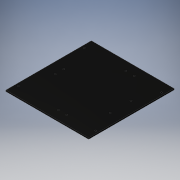
# Autodesk Inventor part: BottomPlate
Saved by Autodesk Inventor 2016 (Build 200138000, 138)
## iProperties
Created: 2015-08-28
Part Number: BottomPlate
Material: Generic
Document SubType Name: Modeling
Designer: lachesis
Density: 1 g/cm^3
Appearance: Glossy - Black
Author: lachesis
Autodesk Inventor part; units mm, degrees
ref_plane "YZ Plane" through (0, 0, 0) normal (1, 0, 0) x (0, 1, 0)
ref_plane "XZ Plane" through (0, 0, 0) normal (0, 1, 0) x (-1, 0, 0)
ref_plane "XY Plane" through (0, 0, 0) normal (0, 0, 1) x (1, 0, 0)
sketch "Block1" plane through (0, 0, 0) normal (0, 0, 1) x (1, 0, 0)
  circle A0 centre (244.9891, 313.0766) radius 1.651
  circle A1 centre (305.4278, 286.7035) radius 1.651
  circle A2 centre (242.5353, 295.4667) radius 1.651
  circle A3 centre (307.8815, 304.3134) radius 1.651
  circle A4 centre (325.7478, 277.8135) radius 1.651
  circle A5 centre (227.9578, 277.8135) radius 1.651
  circle A6 centre (194.5568, 203.1375) radius 1.651
  circle A7 centre (325.7478, 166.5615) radius 1.651
  circle A8 centre (227.9578, 166.5615) radius 1.651
  circle A9 centre (247.0078, 166.5615) radius 1.651
  circle A10 centre (344.7978, 166.5615) radius 1.651
  circle A11 centre (194.5568, 241.2375) radius 1.651
  circle A12 centre (247.0078, 277.8135) radius 1.651
  circle A13 centre (344.7978, 277.8135) radius 1.651
  circle A14 centre (181.8568, 156.6555) radius 1.905
  circle A15 centre (181.8568, 312.8401) radius 1.905
  circle A16 centre (365.194, 312.8401) radius 1.905
  circle A17 centre (365.194, 156.6555) radius 1.905
  line L0 (371.544, 133.5415) -> (371.544, 335.9541)
  line L1 (175.5068, 133.5415) -> (371.544, 133.5415)
  line L2 (175.5068, 335.9541) -> (175.5068, 133.5415)
  line L3 (371.544, 335.9541) -> (175.5068, 335.9541)
  point P0 (271.6644, 239.9388)
sketch "Sketch2" plane through (0, 0, 0) normal (0, 1, 0) x (-1, 0, 0)
  line L0 (98.0186, -101.2063) -> (-98.0186, -101.2063)
  line L1 (-98.0186, -101.2063) -> (-98.0186, 101.2063)
  line L2 (-98.0186, 101.2063) -> (98.0186, 101.2063)
  line L3 (98.0186, 101.2063) -> (98.0186, -101.2063)
  point P0 (0, 0)
  point P1 (-98.0186, 0)
  point P2 (0, -101.2063)
  dimension "d2" = 202.4126
  dimension "d3" = 196.0372
  constraints: 8 end point, 2 midpoint, 2 parallel, 1 horizontal, 1 horizontal alignment, 1 perpendicular, 1 vertical alignment
  measures "d2" distance of L0.end L1.end
  measures "d3" distance of L0.start L0.end
extrude "Extrusion2" add sketch "Sketch2" along normal blind 3
sketch "Sketch3" plane through (0, 3, 0) normal (0, 1, 0) x (1, 0, 0)
  line L0 (98.0186, 101.2063) -> (-98.0186, 101.2063) projected
  line L1 (-98.0186, 101.2063) -> (-98.0186, -101.2063) projected
  line L2 (98.0186, -101.2063) -> (98.0186, 101.2063) projected
  line L3 (-98.0186, -101.2063) -> (98.0186, -101.2063) projected
  line L4 (98.0186, 0) -> (-98.0186, 0) construction
  line L5 (72.3138, 24.765) -> (98.0186, 24.765) construction
  line L6 (-72.3138, 10.1219) -> (-98.0186, 10.1219) construction
  point P0 (0, 0)
  point P1 (-91.6686, 78.0923)
  point P2 (91.6686, 78.0923)
  point P3 (-91.6686, -78.0923)
  point P4 (91.6686, -78.0923)
  point P5 (5.0038, 80.01)
  point P6 (24.9113, 80.01)
  point P7 (72.3138, -24.765)
  point P8 (5.0038, -80.01)
  point P9 (24.9113, -80.01)
  point P10 (-72.3138, -10.1219)
  dimension "d6" = 23.114
  dimension "d7" = 6.35
  dimension "d8" = 23.114
  dimension "d9" = 6.35
  dimension "d10" = 23.114
  dimension "d11" = 6.35
  dimension "d12" = 6.35
  dimension "d13" = 23.114
  dimension "d24" = 19.9075
  dimension "d25" = 49.53
  dimension "d26" = 72.7943
  dimension "d27" = 72.7943
  dimension "d28" = 24.765
  dimension "d29" = 160.02
  dimension "d31" = 20.2438
  dimension "d32" = 10.1219
  dimension "d33" = 144.6276
  constraints: 6 end point, 4 vertical alignment, 2 horizontal alignment, 2 midpoint, 2 perpendicular, 2 point on line, 1 parallel
  measures "d6" distance from line of L0 point (-91.669, 78.092)
  measures "d7" distance from line of L1 point (-91.669, 78.092)
  measures "d8" distance from line of L0 point (91.669, 78.092)
  measures "d9" distance from line of L2 point (91.669, 78.092)
  measures "d10" distance from line of L3 point (-91.669, -78.092)
  measures "d11" distance from line of L1 point (-91.669, -78.092)
  measures "d12" distance from line of L2 point (91.669, -78.092)
  measures "d13" distance from line of L3 point (91.669, -78.092)
  measures "d24" distance of point (24.911, 80.01) point (5.004, 80.01)
  measures "d25" distance of point (72.314, -24.765) L5.start
  measures "d26" distance of point (24.911, 80.01) L5.start
  measures "d27" distance of point (72.314, -24.765) point (24.911, -80.01)
  measures "d28" distance from line of L4 L5.start
  measures "d29" distance of point (5.004, -80.01) point (5.004, 80.01)
  measures "d31" distance of point (-72.314, -10.122) L6.start
  measures "d32" distance from line of L4 point (-72.314, -10.122)
  measures "d33" horizontal distance of L5.start L6.start
hole "Hole1" at (-91.6686, 3, -78.0923) at (91.6686, 3, -78.0923) at (-91.6686, 3, 78.0923) at (91.6686, 3, 78.0923) at (5.0038, 3, -80.01) at (24.9113, 3, -80.01) at (72.3138, 3, -24.765) at (72.3138, 3, 24.765) at (5.0038, 3, 80.01) at (24.9113, 3, 80.01) at (-72.3138, 3, -10.1219) at (-72.3138, 3, 10.1219) direction (0, -1, 0) diameter 3.81 end through all
equation "\"d8\" = d6"
equation "\"d9\" = d7"
equation "\"d10\" = d6"
equation "\"d11\" = d7"
equation "\"d12\" = d7"
equation "\"d13\" = d6"
equation "\"d27\" = d26"
equation "\"d28\" = 0.5 * d25"
equation "\"d32\" = 0.5 * d31"
body "Solid2"
